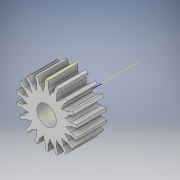
# Autodesk Inventor part: cog_index
Saved by Autodesk Inventor 2018 (Build 220112000, 112)
## iProperties
Created: 2018-02-08
Part Number: cog_index
Material: Generic
Document SubType Name: Modeling
Designer: rheal
Density: 1 g/cm^3
Appearance: Default
Author: rheal
Autodesk Inventor part; units mm, degrees
ref_plane "YZ Plane" through (0, 0, 0) normal (1, 0, 0) x (0, 1, 0)
ref_plane "XZ Plane" through (0, 0, 0) normal (0, 1, 0) x (-1, 0, 0)
ref_plane "XY Plane" through (0, 0, 0) normal (0, 0, 1) x (1, 0, 0)
sketch "Sketch1" plane through (0, 0, 0) normal (0, 0, 1) x (1, 0, 0)
  circle A0 centre (0, 0) radius 3.125
  circle A1 centre (0, 0) radius 1.625
  dimension "d0" = 6.25
  dimension "d1" = 3.25
  constraints: 2 centre point, 2 coincident
  measures "d0" diameter of A0
  measures "d1" diameter of A1
extrude "Extrusion1" add sketch "Sketch1" along normal blind 5
sketch "Sketch2" plane through (0, 0, 5) normal (0, 0, 1) x (1, 0, 0)
  circle A0 centre (0, 0) radius 3.125 projected
  line L0 (0, 3.125) -> (0, 5.125)
  line L1 (-0.25, 3.125) -> (0.25, 3.125)
  line L2 (0.25, 3.125) -> (0.25, 5.125)
  line L3 (0.25, 5.125) -> (-0.25, 5.125)
  line L4 (-0.25, 5.125) -> (-0.25, 3.125)
  line L5 (-0.25, 3.125) -> (0.25, 5.125) construction
  line L6 (0.25, 3.125) -> (-0.25, 5.125) construction
  line L7 (0, 3.125) -> (0, 2.625)
  line L8 (0, 2.625) -> (0.6, 2.625)
  arc A1 (0.6, 2.625) -> (0.25, 4.125) centre (-2.3986, 2.7162) ccw
  line L9 (0, 2.625) -> (-0.6, 2.625)
  arc A2 (-0.25, 4.125) -> (-0.6, 2.625) centre (2.3986, 2.7162) ccw
  point P0 (0, 4.125)
  point P1 (-1, 2.625)
  dimension "d4" = 2
  dimension "d5" = 0.5
  dimension "d6" = 0.5
  dimension "d7" = 0.6
  dimension "d8" = 1.6
  dimension "d10" = 3
  dimension "d18" = 0.6
  dimension "d19" = 3
  constraints: 20 end point, 5 midpoint, 4 point on circle, 3 perpendicular, 2 centre point, 2 horizontal, 2 parallel, 1 point on line, 1 vertical, 1 vertical alignment, 1 other
  measures "d4" distance of L0.start L0.end
  measures "d5" distance of L3.end L2.end
  measures "d6" distance of L0.start L7.end
  measures "d7" distance of L7.end L8.end
  measures "d8" distance of L8.end point (-1, 2.625)
  measures "d10" radius of A1
  measures "d18" distance of L7.end L9.end
  measures "d19" radius of A2
extrude "Extrusion2" add sketch "Sketch2" against normal blind 5 contours A1 L8 L7 A0 | A0 L1 L2 A1 | A2 L4 L1 A0 | A0 L7 L9 A2 | L1 L4 L3 L0 | L0 L3 L2 L1
ref_plane "Work Plane1" through (0, 4.125, 5) normal (1, 0, 0) x (0, 0, -1)
sketch "Sketch3" plane through (0, 4.125, 5) normal (1, 0, 0) x (0, 0, -1)
  line L0 (5, -4.125) -> (9.15, -4.125)
  constraints: 2 end point, 1 horizontal
pattern_circular "Circular Pattern1" count 18 over 360 about axis through (0, 0, 0) along (0, 0, -1) of "Extrusion2"
body "Solid1"
